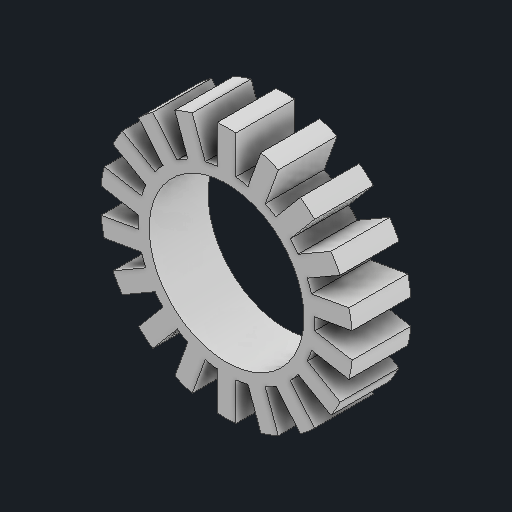
# Autodesk Inventor part: Dummy_Stator
Saved by Autodesk Inventor 2025.1 (Build 291241020, 241B)
## iProperties
Created: 2025-07-24
Part Number: Dummy_Stator
Material: 일반
Document SubType Name: Modeling
Designer: acalo
Density: 1 g/cm^3
Appearance: 기본값
Author: acalo
Autodesk Inventor part; units mm, degrees
ref_plane "YZ Plane" through (0, 0, 0) normal (1, 0, 0) x (0, 1, 0)
ref_plane "XZ Plane" through (0, 0, 0) normal (0, 1, 0) x (-1, 0, 0)
ref_plane "XY Plane" through (0, 0, 0) normal (0, 0, 1) x (1, 0, 0)
sketch "스케치1" plane through (0, 0, 0) normal (0, 0, 1) x (1, 0, 0)
  circle A0 centre (0, 0) radius 18.4
  arc A1 (2.2, 29.9192) -> (-2.2, 29.9192) centre (0, 0) ccw
  arc A2 (-2.2, 20.8844) -> (2.2, 20.8844) centre (0, 0) ccw
  line L0 (2.2, 29.9192) -> (-2.2, 29.9192)
  line L1 (-2.2, 29.9192) -> (-2.2, 20.8844)
  line L2 (2.2, 20.8844) -> (2.2, 29.9192)
  arc A3 (-8.1657, 28.8673) -> (-12.3003, 27.3624) centre (0, 0) ccw
  line L3 (-8.1657, 28.8673) -> (-12.3003, 27.3624)
  line L4 (-12.3003, 27.3624) -> (-9.2102, 18.8725)
  line L5 (-5.0756, 20.3774) -> (-8.1657, 28.8673)
  arc A4 (-17.5464, 24.3336) -> (-20.917, 21.5053) centre (0, 0) ccw
  line L6 (-17.5464, 24.3336) -> (-20.917, 21.5053)
  line L7 (-20.917, 21.5053) -> (-15.1096, 14.5843)
  line L8 (-11.739, 17.4125) -> (-17.5464, 24.3336)
  arc A5 (-24.8108, 16.8649) -> (-27.0108, 13.0544) centre (0, 0) ccw
  line L9 (-24.8108, 16.8649) -> (-27.0108, 13.0544)
  line L10 (-27.0108, 13.0544) -> (-19.1865, 8.537)
  line L11 (-16.9865, 12.3475) -> (-24.8108, 16.8649)
  arc A6 (-29.0827, 7.362) -> (-29.8467, 3.0288) centre (0, 0) ccw
  line L12 (-29.0827, 7.362) -> (-29.8467, 3.0288)
  line L13 (-29.8467, 3.0288) -> (-20.9492, 1.46)
  line L14 (-20.1851, 5.7931) -> (-29.0827, 7.362)
  arc A7 (-29.8467, -3.0288) -> (-29.0827, -7.362) centre (0, 0) ccw
  line L15 (-29.8467, -3.0288) -> (-29.0827, -7.362)
  line L16 (-29.0827, -7.362) -> (-20.1851, -5.7931)
  line L17 (-20.9492, -1.46) -> (-29.8467, -3.0288)
  arc A8 (-27.0108, -13.0544) -> (-24.8108, -16.8649) centre (0, 0) ccw
  line L18 (-27.0108, -13.0544) -> (-24.8108, -16.8649)
  line L19 (-24.8108, -16.8649) -> (-16.9865, -12.3475)
  line L20 (-19.1865, -8.537) -> (-27.0108, -13.0544)
  arc A9 (-20.917, -21.5053) -> (-17.5464, -24.3336) centre (0, 0) ccw
  line L21 (-20.917, -21.5053) -> (-17.5464, -24.3336)
  line L22 (-17.5464, -24.3336) -> (-11.739, -17.4125)
  line L23 (-15.1096, -14.5843) -> (-20.917, -21.5053)
  arc A10 (-12.3003, -27.3624) -> (-8.1657, -28.8673) centre (0, 0) ccw
  line L24 (-12.3003, -27.3624) -> (-8.1657, -28.8673)
  line L25 (-8.1657, -28.8673) -> (-5.0756, -20.3774)
  line L26 (-9.2102, -18.8725) -> (-12.3003, -27.3624)
  arc A11 (-2.2, -29.9192) -> (2.2, -29.9192) centre (0, 0) ccw
  line L27 (-2.2, -29.9192) -> (2.2, -29.9192)
  line L28 (2.2, -29.9192) -> (2.2, -20.8844)
  line L29 (-2.2, -20.8844) -> (-2.2, -29.9192)
  arc A12 (8.1657, -28.8673) -> (12.3003, -27.3624) centre (0, 0) ccw
  line L30 (8.1657, -28.8673) -> (12.3003, -27.3624)
  line L31 (12.3003, -27.3624) -> (9.2102, -18.8725)
  line L32 (5.0756, -20.3774) -> (8.1657, -28.8673)
  arc A13 (17.5464, -24.3336) -> (20.917, -21.5053) centre (0, 0) ccw
  line L33 (17.5464, -24.3336) -> (20.917, -21.5053)
  line L34 (20.917, -21.5053) -> (15.1096, -14.5843)
  line L35 (11.739, -17.4125) -> (17.5464, -24.3336)
  arc A14 (24.8108, -16.8649) -> (27.0108, -13.0544) centre (0, 0) ccw
  line L36 (24.8108, -16.8649) -> (27.0108, -13.0544)
  line L37 (27.0108, -13.0544) -> (19.1865, -8.537)
  line L38 (16.9865, -12.3475) -> (24.8108, -16.8649)
  arc A15 (29.0827, -7.362) -> (29.8467, -3.0288) centre (0, 0) ccw
  line L39 (29.0827, -7.362) -> (29.8467, -3.0288)
  line L40 (29.8467, -3.0288) -> (20.9492, -1.46)
  line L41 (20.1851, -5.7931) -> (29.0827, -7.362)
  arc A16 (29.8467, 3.0288) -> (29.0827, 7.362) centre (0, 0) ccw
  line L42 (29.8467, 3.0288) -> (29.0827, 7.362)
  line L43 (29.0827, 7.362) -> (20.1851, 5.7931)
  line L44 (20.9492, 1.46) -> (29.8467, 3.0288)
  arc A17 (27.0108, 13.0544) -> (24.8108, 16.8649) centre (0, 0) ccw
  line L45 (27.0108, 13.0544) -> (24.8108, 16.8649)
  line L46 (24.8108, 16.8649) -> (16.9865, 12.3475)
  line L47 (19.1865, 8.537) -> (27.0108, 13.0544)
  arc A18 (20.917, 21.5053) -> (17.5464, 24.3336) centre (0, 0) ccw
  line L48 (20.917, 21.5053) -> (17.5464, 24.3336)
  line L49 (17.5464, 24.3336) -> (11.739, 17.4125)
  line L50 (15.1096, 14.5843) -> (20.917, 21.5053)
  arc A19 (12.3003, 27.3624) -> (8.1657, 28.8673) centre (0, 0) ccw
  line L51 (12.3003, 27.3624) -> (8.1657, 28.8673)
  line L52 (8.1657, 28.8673) -> (5.0756, 20.3774)
  line L53 (9.2102, 18.8725) -> (12.3003, 27.3624)
  dimension "d6" = 360
  constraints: 108 end point, 36 point on circle, 19 centre point, 2 coincident, 2 perpendicular, 167 other
extrude "돌출1" add sketch "스케치1" along normal blind 14
